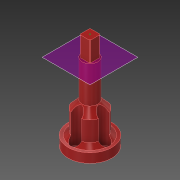
# Autodesk Inventor part: CH_01_0009_servo_shaft
Saved by Autodesk Inventor 2022 (Build 260153000, 153)
## iProperties
Created: 2022-02-25
Part Number: CH_01_0009_servo_shaft
Material: Generic
Document SubType Name: Modeling
Designer: Tomasz Krakowski
Density: 1 g/cm^3
Appearance: Czerwona
Author: Tomasz Krakowski
Autodesk Inventor part; units mm, degrees
ref_plane "YZ Plane" through (0, 0, 0) normal (1, 0, 0) x (0, 1, 0)
ref_plane "XZ Plane" through (0, 0, 0) normal (0, 1, 0) x (-1, 0, 0)
ref_plane "XY Plane" through (0, 0, 0) normal (0, 0, 1) x (1, 0, 0)
sketch "Sketch1" plane through (0, 0, 0) normal (0, 1, 0) x (-1, 0, 0)
  circle A0 centre (0, 0) radius 11
  dimension "d0" = 22
  constraints: 1 centre point, 1 coincident
  measures "d0" diameter of A0
extrude "Extrusion1" add sketch "Sketch1" along normal blind 4.65
sketch "Sketch2" plane through (0, 4.65, 0) normal (0, 1, 0) x (1, 0, 0)
  circle A0 centre (0, 0) radius 4
  dimension "d3" = 8
  constraints: 1 centre point, 1 coincident
  measures "d3" diameter of A0
extrude "Extrusion2" add sketch "Sketch2" along normal blind 44.05
sketch "Szkic4" plane through (0, 4.65, 0) normal (0, 1, 0) x (1, 0, 0)
  circle A0 centre (0, 0) radius 7.5
  dimension "d21" = 15
  constraints: 1 centre point, 1 coincident
  measures "d21" diameter of A0
extrude "Wyciągnięcie proste3" add sketch "Szkic4" along normal blind 12
sketch "Sketch3" plane through (0, 4.65, 0) normal (0, 1, 0) x (1, 0, 0)
  circle A0 centre (0, 0) radius 7 construction
  line L0 (0, 0) -> (-7, 0) construction
  point P0 (0, -7)
  point P1 (7, 0)
  point P2 (0, 7)
  dimension "d6" = 14
  dimension "d9" = 360
  constraints: 2 end point, 1 coincident, 1 horizontal, 1 horizontal alignment, 7 other
hole "Hole1" at (-7, 4.65, 0) at (0, 4.65, 7) at (7, 4.65, 0) at (0, 4.65, -7) direction (0, -1, 0) diameter 3.5 end up to surface start extended yes counterbore diameter 5.5 counterbore depth 3
chamfer "Faza2" distance 2 angle 45 4 edges at (5.3033, 4.65, 5.3033) (-5.3033, 4.65, 5.3033) (5.3033, 4.65, -5.3033) (-5.3033, 4.65, -5.3033)
sketch "Sketch5" plane through (0, 48.7, 0) normal (0, 1, 0) x (1, 0, 0)
  point P0 (0, 0)
ref_plane "Work Plane1" through (0, 38.7, 0) normal (0, -1, 0) x (1, 0, 0)
sketch "Sketch6" plane through (0, 38.7, 0) normal (0, -1, 0) x (1, 0, 0)
  circle A0 centre (0, 0) radius 4 projected
  circle A1 centre (0, 0) radius 4 construction
  line L0 (2.15, 2.65) -> (-2.15, 2.65)
  line L1 (-2.65, 2.15) -> (-2.65, -2.15)
  line L2 (-2.15, -2.65) -> (2.15, -2.65)
  line L3 (2.65, -2.15) -> (2.65, 2.15)
  line L4 (2.65, 2.65) -> (-2.65, -2.65) construction
  line L5 (-2.65, 2.65) -> (2.65, -2.65) construction
  line L6 (-2.15, 2.65) -> (-2.65, 2.15)
  line L7 (-2.65, -2.15) -> (-2.15, -2.65)
  line L8 (2.15, -2.65) -> (2.65, -2.15)
  line L9 (2.65, 2.15) -> (2.15, 2.65)
  dimension "d33" = 5.3
  dimension "d34" = 0.5
  dimension "d35" = 0.5
  dimension "d36" = 0.5
  dimension "d37" = 0.5
  dimension "d38" = 0.5
  dimension "d39" = 0.5
  dimension "d40" = 0.5
  dimension "d41" = 0.5
  constraints: 20 end point, 8 point on line, 2 midpoint, 2 parallel, 2 perpendicular, 1 centre point, 1 coincident, 1 concentric, 1 horizontal
  measures "d33" distance of L5.start L4.end
  measures "d34" distance of L0.end L5.start
  measures "d35" distance of L1.start L5.start
  measures "d36" distance of L1.end L4.end
  measures "d37" distance of L2.start L4.end
  measures "d38" distance of L2.end L5.end
  measures "d39" distance of L3.start L5.end
  measures "d40" distance of L3.end L4.start
  measures "d41" distance of L0.start L4.start
extrude "Extrusion4" cut sketch "Sketch6" against normal through all
chamfer "Chamfer4" distance 3.5 angle 45 1 edges at (-4, 16.65, 0)
equation "\"d35\" = d34"
equation "\"d36\" = d34"
equation "\"d37\" = d36"
equation "\"d38\" = d34"
equation "\"d39\" = d38"
equation "\"d40\" = d34"
equation "\"d41\" = d40"
body "Solid1"
